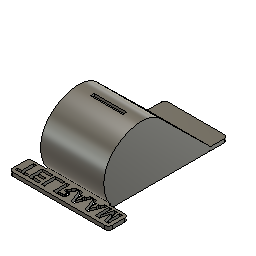
telraam_camera_holder_V1 (Autodesk Fusion 360 design; units mm, degrees)
Autodesk Fusion 360 part; units mm, degrees
note: some values were not read from the file. Chosen so that the rebuilt part matches the saved one: which bodies a step acts on; which face or edge a step refers to. Set by a fixed rule: which sketch regions a step uses.
sketch "Sketch1" plane through (0, 0, 0) normal (0, 1, 0) x (1, 0, 0)
  line L0 (0, 0) -> (30, 0)
  line L1 (30, 0) -> (30, 22)
  line L2 (30, 22) -> (0, 22)
  line L3 (0, 22) -> (0, 0)
  line L4 (0, 22) -> (2.25, 22) construction
  line L5 (2.25, 22) -> (2.25, 19.4) construction
  line L6 (2.25, 19.4) -> (0, 19.4) construction
  line L7 (0, 19.4) -> (0, 22) construction
  line L8 (2.25, 19.4) -> (27.75, 19.4)
  line L9 (27.75, 19.4) -> (27.75, -5)
  line L10 (27.75, -5) -> (2.25, -5)
  line L11 (2.25, -5) -> (2.25, 19.4)
  line L12 (15, -5) -> (15, 0) construction
  line L13 (15, 0) -> (22, 0) construction
  line L14 (22, 0) -> (8, 0)
  line L15 (8, 0) -> (8, 17.5)
  line L16 (8, 17.5) -> (22, 17.5)
  line L17 (22, 17.5) -> (22, 0)
  line L18 (30, 0) -> (0, 0)
  line L19 (0, 0) -> (0, -10)
  line L20 (0, -10) -> (30, -10)
  line L21 (30, -10) -> (30, 0)
  dimension "d1" = 30
  dimension "d2" = 22
  dimension "d3" = 2.25
  dimension "d4" = 2.6
  dimension "d5" = 25.5
  dimension "d6" = 24.4
  dimension "d7" = 5
  dimension "d8" = 7
  dimension "d9" = 14
  dimension "d10" = 17.5
  constraint horizontal L0
  constraint vertical L1
  constraint horizontal L2
  constraint vertical L3
  constraint coincident L0.start L3.end
  constraint horizontal L4
  constraint vertical L5
  constraint horizontal L6
  constraint vertical L7
  constraint horizontal L8
  constraint vertical L9
  constraint horizontal L10
  constraint vertical L11
  constraint midpoint L10 L12.start
  constraint perpendicular L10 L12
  constraint perpendicular L12 L13
  constraint horizontal L14
  constraint vertical L15
  constraint horizontal L16
  constraint vertical L17
  constraint horizontal L18
  constraint vertical L19
  constraint horizontal L20
  constraint vertical L21
  measures "d1" distance of L0.start L0.end
  measures "d2" distance of L0.start L2.end
  measures "d3" distance of L2.end L4.end
  measures "d4" distance of L2.end L6.end
  measures "d5" distance of L5.end L8.end
  measures "d6" distance of L5.end L10.end
  measures "d7" distance of L12.start L12.end
  measures "d8" distance of L12.end L13.end
  measures "d9" distance of L13.end L14.end
  measures "d10" distance of L13.end L16.end
extrude "Extrude1" add sketch "Sketch1" along normal blind 10 contours L0 L9 L10 L11 L18 L19 L20 L21 | L0 L1 L2 L3 L8 L9 L11 L18 makes body 1
extrude "Extrude2" add sketch "Sketch1" along normal blind 8 contours L0 L9 L10 L11 L14 L18 | L0 L8 L9 L11 L15 L16 L17 L18 bodies 1
sketch "Sketch2" plane through (0, 10, 0) normal (0, 1, 0) x (-1, 0, 0)
  line L0 (-27.75, 5) -> (-2.25, 5)
  line L1 (-2.25, 5) -> (-2.25, -19.4)
  line L2 (-2.25, -19.4) -> (-27.75, -19.4)
  line L3 (-27.75, -19.4) -> (-27.75, 5)
  line L4 (-30, 10) -> (-30, -22)
  line L5 (-30, -22) -> (0, -22)
  line L6 (0, -22) -> (0, 10)
  line L7 (0, 10) -> (-30, 10)
  line L8 (-15, 5) -> (-23.4414, 5) construction
  line L9 (-23.4414, 5) -> (-6.4414, 5)
  line L10 (-6.4414, 5) -> (-6.4414, 18)
  line L11 (-6.4414, 18) -> (-23.4414, 18)
  line L12 (-23.4414, 18) -> (-23.4414, 5)
  dimension "d15" = 17
  constraint midpoint L0 L8.start
  constraint coincident L0 L8.end
  constraint parallel L0 L8
  constraint horizontal L9
  constraint vertical L10
  constraint horizontal L11
  constraint vertical L12
  measures "d15" distance of L8.end L9.end
extrude "Extrude3" cut sketch "Sketch2" against normal blind 1 contours L0 L7 L9 L10 L12 bodies 1
sketch "Sketch5" plane through (0, 0, 0) normal (-1, 0, 0) x (0, 0, 1)
  line L0 (-22, 0) -> (10, 0)
  line L1 (10, 0) -> (10, 10)
  line L2 (10, 10) -> (-22, 10)
  line L3 (-22, 10) -> (-22, 0)
  line L4 (10, 10) -> (-22, 10)
  line L5 (10, 0) -> (10, 10)
  line L6 (-22, 0) -> (-22, 10)
  line L7 (10, 0) -> (-22, 0)
  line L8 (10, 5) -> (5, 5) construction
  circle A0 centre (5, 5) radius 5
  circle A1 centre (5, 5) radius 3
  dimension "d31" = 5
  dimension "d32" = 6
  constraint midpoint L1 L8.start
  constraint perpendicular L1 L8
  constraint coincident L8.end A0.centre
  constraint coincident L8.start A0
  constraint concentric A0 A1
  measures "d31" distance of L8.start L8.end
  measures "d32" diameter of A1
extrude "Extrude5" cut sketch "Sketch5" against normal blind 30 contours A1 bodies 1
extrude "Extrude6" cut sketch "Sketch5" against normal blind 30 contours L0 L1 L5 L7 A0 | L1 L2 L4 L5 A0 bodies 1
sketch "Sketch10" plane through (30, 0, 0) normal (1, 0, 0) x (0, 0, -1)
  arc A0 (-5, 10) -> (-5, 0) centre (-5, 5) ccw
  line L0 (-5, 0) -> (22, 0)
  line L1 (22, 0) -> (22, 10)
  line L2 (22, 10) -> (-5, 10)
  circle A1 centre (-5, 5) radius 3
  arc A2 (-5, 10) -> (-5, 0) centre (-5, 5) ccw
  circle A3 centre (-5, 5) radius 3
  line L3 (22, 10) -> (-5, 10)
  line L4 (22, 0) -> (22, 10)
  line L5 (22, 0) -> (-5, 0)
  circle A4 centre (-5, 5) radius 2.75
  circle A5 centre (-5, 5) radius 28 construction
  line L6 (-5, 5) -> (16.3152, 26.3152) construction
  line L7 (-5, 5) -> (25.7881, 5) construction
  line L8 (14.799, 24.799) -> (11.2635, 28.3345) construction
  line L9 (11.2635, 28.3345) -> (39.6303, -0.0323)
  line L10 (39.6303, -0.0323) -> (49.6303, -0.0323)
  spline S0 degree 5 poles (11.2635, 28.3345) (10.5414, 28.9553) (9.0442, 30.055) (6.6392, 31.2791) (3.1553, 32.0787) (-1.4187, 31.8066) (-5.8903, 30.427) (-9.919, 28.1364) (-13.2046, 25.151) (-15.548, 21.6967) (-16.9173, 18.001) (-17.397, 14.2819) (-17.1414, 10.738) (-16.3304, 7.5364) (-15.1311, 4.8024) (-13.6528, 2.6017) (-12.2918, 1.2849) (-11.1808, 0.5463) (-10.4002, 0.1638) (-10, 0) knots 0 0 0 0 0 0 0.066667 0.133333 0.2 0.266667 0.333333 0.4 0.466667 0.533333 0.6 0.666667 0.733333 0.8 0.866667 0.933333 1 1 1 1 1 1
  line L11 (15.5269, 24.669) -> (7, 32)
  spline S1 degree 5 poles (11.4377, 30.0185) (10.7333, 30.6009) (9.2645, 31.631) (6.8809, 32.7721) (3.3818, 33.5028) (-1.2891, 33.2032) (-5.9391, 31.8407) (-10.2242, 29.5954) (-13.8317, 26.6674) (-16.5299, 23.2679) (-18.243, 19.6138) (-19.051, 15.9194) (-19.1227, 12.3855) (-18.6719, 9.1891) (-17.9107, 6.4719) (-17.0026, 4.3263) (-16.2218, 3.0932) (-15.6179, 2.4413) (-15.2073, 2.127) (-15, 2) knots 0 0 0 0 0 0 0.066667 0.133333 0.2 0.266667 0.333333 0.4 0.466667 0.533333 0.6 0.666667 0.733333 0.8 0.866667 0.933333 1 1 1 1 1 1
  line L12 (15.4746, 26.6807) -> (7.4008, 33.3564)
  line L13 (-10, 0) -> (-25, 0)
  line L14 (-25, 0) -> (-25, 2)
  line L15 (-25, 2) -> (-15, 2)
  line L16 (49.6303, -0.0323) -> (49.6303, 1.9677)
  line L17 (49.6303, 1.9677) -> (40, 1.9677)
  line L18 (40, 1.9677) -> (11.4377, 30.0185)
  line L19 (-10, 0) -> (39.6303, -0.0323)
  point P0 (-13, 25)
  point P1 (-16, 7)
  point P2 (-15, 25)
  point P3 (-18, 7)
  dimension "d59" = 5.5
  dimension "d60" = 56
  dimension "d61" = 45
  dimension "d62" = 5
  dimension "d63" = 10
  dimension "d64" = 2
  constraint concentric A2 A4
  constraint concentric A4 A5
  constraint horizontal L7
  constraint coincident A0.centre A1.centre
  constraint coincident A5 L8.start
  constraint coincident L6 L8.start
  constraint perpendicular L6 L8
  constraint perpendicular L6 L9
  constraint horizontal L10
  constraint midpoint L8.end L11
  constraint midpoint S1.start L12
  constraint horizontal L13
  constraint perpendicular L13 L14
  constraint perpendicular L14 L15
  constraint perpendicular L10 L16
  constraint perpendicular L16 L17
  measures "d59" diameter of A4
  measures "d60" diameter of A5
  measures "d61" angle of L6 L7
  measures "d62" distance of L8.start L8.end
  measures "d63" distance of L9.end L10.end
  measures "d64" distance of L10.end L16.end
extrude "Extrude10" add sketch "Sketch10" along normal blind 2 from surface at 0.5 separate body contours A0 L0 L1 L2 A2 L3 L4 L5 | A1 A3 | A4 | L9 L10 S0 S1 L13 L14 L15 L16 L17 L18 | L9 S0 L19 makes body 2
extrude "Extrude11" add sketch "Sketch10" along normal blind -27 and the other way blind -1 contours A4 bodies 2
extrude "Extrude12" add sketch "Sketch10" along normal blind -30.5 and the other way blind -1 contours L9 L10 S0 S1 L13 L14 L15 L16 L17 L18 bodies 2
extrude "Extrude13" add sketch "Sketch10" against normal blind 2 from surface at -30.5 contours A0 L0 L1 L2 A2 L3 L4 L5 | A1 A3 | A4 | L9 L10 S0 S1 L13 L14 L15 L16 L17 L18 | L9 S0 L19 bodies 2
sketch "Sketch11" plane through (-2.5, 0, 0) normal (-1, 0, 0) x (0, 0, 1)
  line L0 (10, 0) -> (25, 0)
  line L1 (25, 0) -> (25, 2)
  line L2 (25, 2) -> (15, 2)
  spline S0 degree 5 poles (15, 2) (15.2073, 2.127) (15.6179, 2.4413) (16.2218, 3.0932) (17.0026, 4.3263) (17.9107, 6.4719) (18.6719, 9.1891) (19.1227, 12.3855) (19.051, 15.9194) (18.243, 19.6138) (16.5299, 23.2679) (13.8317, 26.6674) (10.2242, 29.5954) (5.9391, 31.8407) (1.2891, 33.2032) (-3.3818, 33.5028) (-6.8809, 32.7721) (-9.2645, 31.631) (-10.7333, 30.6009) (-11.4377, 30.0185) knots -1 -1 -1 -1 -1 -1 -0.933333 -0.866667 -0.8 -0.733333 -0.666667 -0.6 -0.533333 -0.466667 -0.4 -0.333333 -0.266667 -0.2 -0.133333 -0.066667 0 0 0 0 0 0
  line L3 (-11.4377, 30.0185) -> (-40, 1.9677)
  line L4 (-40, 1.9677) -> (-49.6303, 1.9677)
  line L5 (-49.6303, 1.9677) -> (-49.6303, -0.0323)
  line L6 (-49.6303, -0.0323) -> (-39.6303, -0.0323)
  line L7 (-39.6303, -0.0323) -> (10, 0)
  arc A0 (5, 0) -> (5, 10) centre (5, 5) ccw
  line L8 (5, 10) -> (-22, 10)
  circle A1 centre (5, 5) radius 3
  line L9 (-22, 0) -> (-22, 10)
  line L10 (5, 0) -> (-22, 0)
  circle A2 centre (5, 5) radius 5.5
  dimension "d79" = 11
  constraint concentric A0 A2
  measures "d79" diameter of A2
extrude "Extrude14" cut sketch "Sketch11" against normal blind 2 contours L7 L10 A2 | L7 A0 L8 A2 | L7 A0 L8 L10 A2 | A1 bodies 2
sketch "Sketch12" plane through (0, 0, 0) normal (-1, 0, 0) x (0, 0, 1)
  circle A0 centre (5, 5) radius 3
  arc A1 (5, 0) -> (5, 10) centre (5, 5) ccw
  line L0 (5, 10) -> (-22, 10)
  line L1 (-22, 10) -> (-22, 0)
  line L2 (-22, 0) -> (5, 0)
  circle A2 centre (5, 5) radius 5
  constraint concentric A0 A2
extrude "Extrude15" add sketch "Sketch12" along normal blind 3 contours A0 | A1 A2 bodies 1
sketch "Sketch13" plane through (-3, 0, 0) normal (-1, 0, 0) x (0, 0, 1)
  circle A0 centre (5, 5) radius 5
  line L0 (5, 0) -> (-22, 0)
  line L1 (-22, 0) -> (-22, 5)
  line L2 (-22, 5) -> (5, 5)
  line L3 (5, 5) -> (5, 0)
  constraint horizontal L0
  constraint vertical L1
  constraint horizontal L2
  constraint vertical L3
  constraint coincident A0 L0.start
extrude "Extrude16" add sketch "Sketch13" along normal blind 3 bodies 1
sketch "Sketch14" plane through (0, 0, 5) normal (0, 0, -1) x (-1, 0, 0)
  line L0 (-23.4414, 9) -> (-23.4414, 10)
  line L1 (-23.4414, 10) -> (-27.75, 10)
  line L2 (-27.75, 10) -> (-27.75, 8)
  line L3 (-27.75, 8) -> (-2.25, 8)
  line L4 (-2.25, 8) -> (-2.25, 10)
  line L5 (-2.25, 10) -> (-6.4414, 10)
  line L6 (-6.4414, 10) -> (-6.4414, 9)
  line L7 (-6.4414, 9) -> (-23.4414, 9)
  line L8 (-27.75, 10) -> (-26.8336, 10)
  line L9 (-26.8336, 10) -> (-26.8336, 9.2)
  line L10 (-26.8336, 9.2) -> (-27.75, 9.2)
  line L11 (-27.75, 9.2) -> (-27.75, 10)
  line L12 (-2.25, 10) -> (-3.1585, 10)
  line L13 (-3.1585, 10) -> (-3.1585, 9.2)
  line L14 (-3.1585, 9.2) -> (-2.25, 9.2)
  line L15 (-2.25, 9.2) -> (-2.25, 10)
  dimension "d88" = 0.8
  dimension "d89" = 0.8
  constraint horizontal L8
  constraint vertical L9
  constraint horizontal L10
  constraint vertical L11
  constraint coincident L1.end L2.start
  constraint horizontal L12
  constraint vertical L13
  constraint horizontal L14
  constraint vertical L15
  constraint coincident L4.end L5.start
  measures "d88" distance of L1.end L10.end
  measures "d89" distance of L4.end L14.end
extrude "Extrude17" add sketch "Sketch14" along normal blind 2 contours L1 L2 L8 L9 L10 L11 | L4 L5 L12 L13 L14 L15 bodies 1
fillet "Fillet5" radius 0.5 4 edges at (3.1585, 9.2, 4) (2.7043, 9.2, 3) (26.8336, 9.2, 4) (27.2918, 9.2, 3) on bodies 1
sketch "Sketch15" plane through (0, 0, -19.4) normal (0, 0, 1) x (1, 0, 0)
  line L0 (2.25, 8) -> (27.75, 8)
  line L1 (27.75, 8) -> (27.75, 10)
  line L2 (27.75, 10) -> (2.25, 10)
  line L3 (2.25, 10) -> (2.25, 8)
  line L4 (9.9542, 10) -> (20.0929, 10)
  line L5 (20.0929, 10) -> (20.0929, 9.2)
  line L6 (20.0929, 9.2) -> (9.9542, 9.2)
  line L7 (9.9542, 9.2) -> (9.9542, 10)
  dimension "d94" = 0.8
  constraint horizontal L4
  constraint vertical L5
  constraint horizontal L6
  constraint vertical L7
  constraint coincident L2 L4.start
  measures "d94" distance of L4.start L6.end
extrude "Extrude18" add sketch "Sketch15" along normal blind 0.4 contours L2 L4 L5 L6 L7 bodies 1
fillet "Fillet6" radius 0.4 2 edges at (15.0235, 10, -19) (15.0235, 9.2, -19) on bodies 1
fillet "Fillet7" radius 4 2 edges at (30, 5, -22) (0, 5, -22) on bodies 1
sketch "Sketch17" plane through (0, 0, 0) normal (0, 1, 0) x (1, 0, 0)
  arc A0 (4, 22) -> (0, 18) centre (4, 18) ccw
  line L0 (26, 22) -> (4, 22)
  arc A1 (30, 18) -> (26, 22) centre (26, 18) ccw
  line L1 (30, -10) -> (30, -5)
  line L2 (30, -5) -> (30, 18)
  line L3 (-3, 0) -> (-3, 22)
  line L4 (-6, 22) -> (-6, -5)
  line L5 (-3, 22) -> (-6, 22)
  line L6 (-6, -5) -> (-6, -10)
  line L7 (0, 18) -> (0, 0)
  line L8 (8, 0) -> (8, 17.5)
  line L9 (22, 0) -> (8, 0)
  line L10 (22, 17.5) -> (22, 0)
  line L11 (8, 17.5) -> (22, 17.5)
  line L12 (-6, -10) -> (30, -10)
  line L13 (-3, 0) -> (0, 0)
  line L14 (6, 0) -> (24, 0)
  line L15 (24, 0) -> (24, 2)
  line L16 (24, 2) -> (6, 2)
  line L17 (6, 2) -> (6, 0)
  constraint horizontal L14
  constraint vertical L15
  constraint horizontal L16
  constraint vertical L17
extrude "Extrude19" cut sketch "Sketch17" along normal blind 37 from surface at 20 contours L8 L14 L16 L17 | L8 L9 L10 L14 L16 | L10 L14 L15 L16 bodies 2
sketch "Sketch18" plane through (0, 0, 0) normal (0, -1, 0) x (1, 0, 0)
  line L0 (-2.5, 25) -> (-2.5, 10)
  line L1 (-2.5, 10) -> (-0.5, 10)
  line L2 (-0.5, 10) -> (30.5, 10)
  line L3 (30.5, 10) -> (32.5, 10)
  line L4 (32.5, 10) -> (32.5, 25)
  line L5 (32.5, 25) -> (-2.5, 25)
  line L6 (-10.5777, 8.9762) -> (41.4223, 8.9762) construction
  line L7 (41.4223, 8.9762) -> (41.4223, 24.9762) construction
  line L8 (41.4223, 24.9762) -> (-10.5777, 24.9762) construction
  line L9 (-10.5777, 24.9762) -> (-10.5777, 8.9762) construction
  line L10 (-12, 16) -> (43, 16)
  line L11 (43, 16) -> (43, 27)
  line L12 (43, 27) -> (-12, 27)
  line L13 (-12, 27) -> (-12, 16)
  line L14 (12.2105, 23.7055) -> (9.3109, 23.7055)
  line L15 (9.3109, 23.7055) -> (9.3109, 21.8124)
  line L16 (9.3109, 21.8124) -> (12.2105, 21.8124)
  line L17 (12.2105, 21.8124) -> (12.2105, 23.7055)
  line L18 (20.5, 20.5) -> (21.6042, 20.5)
  line L19 (21.6042, 20.5) -> (21.6042, 18.745)
  line L20 (21.6042, 18.745) -> (20.5, 18.745)
  line L21 (20.5, 18.745) -> (20.5, 20.5)
  line L22 (28.2661, 20.5) -> (29.3444, 20.5)
  line L23 (29.3444, 20.5) -> (29.3444, 18.745)
  line L24 (29.3444, 18.745) -> (28.2661, 18.745)
  line L25 (28.2661, 18.745) -> (28.2661, 20.5)
  point P0 (15, 25)
  text T0 "TELRAAM" font "Arial" height 7.7 bold align left top in box 52 x 16 at (-10.5777, 8.9762) x (1, 0) y (0, 1) spacing 1
  constraint midpoint L5 P0
  constraint horizontal L10
  constraint vertical L11
  constraint horizontal L12
  constraint vertical L13
  constraint horizontal L14
  constraint vertical L15
  constraint horizontal L16
  constraint vertical L17
  constraint horizontal L18
  constraint vertical L19
  constraint horizontal L20
  constraint vertical L21
  constraint horizontal L22
  constraint vertical L23
  constraint horizontal L24
  constraint vertical L25
extrude "Extrude20" add sketch "Sketch18" against normal blind 2 contours L0 L4 L5 L10 L11 L12 L13 bodies 2
extrude "Extrude22" cut sketch "Sketch18" against normal blind 2 text T0 bodies 2 makes body 3 at (12.6379, 2, 23.0223) makes body 4 at (29.554, 0.6667, 21.275) makes body 5 at (21.7858, 0.6667, 21.275)
sketch "Sketch19" plane through (0, 2, 0) normal (0, 1, 0) x (-1, 0, 0)
  line L0 (-32.5, 16) -> (-32.5, 15)
  line L1 (-32.5, 15) -> (2.5, 15)
  line L2 (2.5, 15) -> (2.5, 16)
  line L3 (2.5, 16) -> (12, 16)
  line L4 (12, 16) -> (12, 27)
  line L5 (12, 27) -> (-43, 27)
  line L6 (-43, 27) -> (-43, 16)
  line L7 (-43, 16) -> (-32.5, 16)
  line L8 (6.7382, 17.2762) -> (6.7382, 23.6736)
  line L9 (6.7382, 23.6736) -> (4.4587, 23.6736)
  line L10 (4.4587, 23.6736) -> (4.4587, 24.9762)
  line L11 (4.4587, 24.9762) -> (10.5777, 24.9762)
  line L12 (10.5777, 24.9762) -> (10.5777, 23.6736)
  line L13 (10.5777, 23.6736) -> (8.2929, 23.6736)
  line L14 (8.2929, 23.6736) -> (8.2929, 17.2762)
  line L15 (8.2929, 17.2762) -> (6.7382, 17.2762)
  line L16 (-9.1818, 17.2762) -> (-9.1818, 18.5735)
  line L17 (-9.1818, 18.5735) -> (-5.316, 18.5735)
  line L18 (-5.316, 18.5735) -> (-5.316, 24.9132)
  line L19 (-5.316, 24.9132) -> (-3.7613, 24.9132)
  line L20 (-3.7613, 24.9132) -> (-3.7613, 17.2762)
  line L21 (-3.7613, 17.2762) -> (-9.1818, 17.2762)
  line L22 (-11.85, 17.2762) -> (-11.85, 20.4906)
  line L23 (-11.85, 20.4906) -> (-12.1651, 20.4906)
  spline S0 degree 3 poles (-12.1651, 20.4906) (-12.3206, 20.4903) (-12.5852, 20.4898) (-12.8418, 20.4272) (-12.9477, 20.4014) knots -0.07901 -0.07901 -0.07901 -0.07901 -0.032603 0 0 0 0
  spline S1 degree 3 poles (-12.9477, 20.4014) (-13.0308, 20.365) (-13.2067, 20.2879) (-13.3432, 20.1525) (-13.4152, 20.081) knots -0.057107 -0.057107 -0.057107 -0.057107 -0.030153 0 0 0 0
  spline S2 degree 3 poles (-13.4152, 20.081) (-13.5219, 19.9495) (-13.8153, 19.5881) (-14.0715, 19.1992) (-14.2346, 18.9517) knots -0.139592 -0.139592 -0.139592 -0.139592 -0.088836 0 0 0 0
  line L24 (-14.2346, 18.9517) -> (-15.3586, 17.2762)
  line L25 (-15.3586, 17.2762) -> (-17.2179, 17.2762)
  line L26 (-17.2179, 17.2762) -> (-16.2778, 18.7784)
  spline S3 degree 3 poles (-16.2778, 18.7784) (-16.1175, 19.0369) (-15.8476, 19.4724) (-15.5223, 19.8678) (-15.3901, 20.0284) knots -0.153464 -0.153464 -0.153464 -0.153464 -0.062342 0 0 0 0
  spline S4 degree 3 poles (-15.3901, 20.0284) (-15.2703, 20.1455) (-15.0181, 20.392) (-14.7178, 20.5772) (-14.5602, 20.6745) knots -0.105457 -0.105457 -0.105457 -0.105457 -0.055357 0 0 0 0
  spline S5 degree 3 poles (-14.5602, 20.6745) (-14.8687, 20.7321) (-15.4392, 20.8386) (-15.8806, 21.212) (-16.0834, 21.3836) knots -0.170594 -0.170594 -0.170594 -0.170594 -0.078353 0 0 0 0
  spline S6 degree 3 poles (-16.0834, 21.3836) (-16.232, 21.5899) (-16.54, 22.0177) (-16.5748, 22.5447) (-16.5929, 22.8175) knots -0.154918 -0.154918 -0.154918 -0.154918 -0.080198 0 0 0 0
  spline S7 degree 3 poles (-16.5929, 22.8175) (-16.5802, 23.0367) (-16.5553, 23.4655) (-16.3548, 23.8452) (-16.2568, 24.0308) knots -0.127215 -0.127215 -0.127215 -0.127215 -0.062196 0 0 0 0
  spline S8 degree 3 poles (-16.2568, 24.0308) (-16.1366, 24.1935) (-15.8993, 24.5149) (-15.5372, 24.6831) (-15.3586, 24.7661) knots -0.117747 -0.117747 -0.117747 -0.117747 -0.058096 0 0 0 0
  spline S9 degree 3 poles (-15.3586, 24.7661) (-15.1176, 24.8269) (-14.5309, 24.9749) (-13.9248, 24.9757) (-13.5675, 24.9762) knots -0.180926 -0.180926 -0.180926 -0.180926 -0.106622 0 0 0 0
  line L27 (-13.5675, 24.9762) -> (-10.2953, 24.9762)
  line L28 (-10.2953, 24.9762) -> (-10.2953, 17.2762)
  line L29 (-10.2953, 17.2762) -> (-11.85, 17.2762)
  line L30 (-29.6871, 24.9762) -> (-28.0431, 24.9762)
  line L31 (-28.0431, 24.9762) -> (-25.044, 17.2762)
  line L32 (-25.044, 17.2762) -> (-26.6932, 17.2762)
  line L33 (-26.6932, 17.2762) -> (-27.3288, 19.0252)
  line L34 (-27.3288, 19.0252) -> (-30.4067, 19.0252)
  line L35 (-30.4067, 19.0252) -> (-31.079, 17.2762)
  line L36 (-31.079, 17.2762) -> (-32.7703, 17.2762)
  line L37 (-32.7703, 17.2762) -> (-29.6871, 24.9762)
  line L38 (-21.9188, 24.9762) -> (-20.2748, 24.9762)
  line L39 (-20.2748, 24.9762) -> (-17.2757, 17.2762)
  line L40 (-17.2757, 17.2762) -> (-18.925, 17.2762)
  line L41 (-18.925, 17.2762) -> (-19.5605, 19.0252)
  line L42 (-19.5605, 19.0252) -> (-22.6384, 19.0252)
  line L43 (-22.6384, 19.0252) -> (-23.3107, 17.2762)
  line L44 (-23.3107, 17.2762) -> (-25.002, 17.2762)
  line L45 (-25.002, 17.2762) -> (-21.9188, 24.9762)
  line L46 (-35.0183, 17.2762) -> (-35.0183, 23.3374)
  line L47 (-35.0183, 23.3374) -> (-36.5415, 17.2762)
  line L48 (-36.5415, 17.2762) -> (-38.0384, 17.2762)
  line L49 (-38.0384, 17.2762) -> (-39.5669, 23.3374)
  line L50 (-39.5669, 23.3374) -> (-39.5669, 17.2762)
  line L51 (-39.5669, 17.2762) -> (-41.0113, 17.2762)
  line L52 (-41.0113, 17.2762) -> (-41.0113, 24.9762)
  line L53 (-41.0113, 24.9762) -> (-38.6792, 24.9762)
  line L54 (-38.6792, 24.9762) -> (-37.2978, 19.7238)
  line L55 (-37.2978, 19.7238) -> (-35.9007, 24.9762)
  line L56 (-35.9007, 24.9762) -> (-33.5739, 24.9762)
  line L57 (-33.5739, 24.9762) -> (-33.5739, 17.2762)
  line L58 (-33.5739, 17.2762) -> (-35.0183, 17.2762)
  line L59 (-2.401, 17.2762) -> (-2.401, 18.5735)
  line L60 (-2.401, 18.5735) -> (1.9007, 18.5735)
  line L61 (1.9007, 18.5735) -> (1.9007, 20.6692)
  line L62 (1.9007, 20.6692) -> (-1.965, 20.6692)
  line L63 (-1.965, 20.6692) -> (-1.965, 21.9666)
  line L64 (-1.965, 21.9666) -> (1.9007, 21.9666)
  line L65 (1.9007, 21.9666) -> (1.9007, 23.6736)
  line L66 (1.9007, 23.6736) -> (-2.2539, 23.6736)
  line L67 (-2.2539, 23.6736) -> (-2.2539, 24.9762)
  line L68 (-2.2539, 24.9762) -> (3.4555, 24.9762)
  line L69 (3.4555, 24.9762) -> (3.4555, 17.2762)
  line L70 (3.4555, 17.2762) -> (-2.401, 17.2762)
  line L71 (-11.85, 21.8295) -> (-13.1477, 21.8295)
  line L72 (-13.1477, 21.8295) -> (-13.1477, 20.3044)
  line L73 (-13.1477, 20.3044) -> (-11.85, 20.3044)
  line L74 (-11.85, 20.3044) -> (-11.85, 21.8295)
  line L75 (-21.6279, 20.4295) -> (-20.5016, 20.4295)
  line L76 (-20.5016, 20.4295) -> (-20.5016, 18.5544)
  line L77 (-20.5016, 18.5544) -> (-21.6279, 18.5544)
  line L78 (-21.6279, 18.5544) -> (-21.6279, 20.4295)
  line L79 (-29.4763, 20.429) -> (-28.3136, 20.429)
  line L80 (-28.3136, 20.429) -> (-28.3136, 19.0252)
  line L81 (-28.3136, 19.0252) -> (-29.4763, 19.0252)
  line L82 (-29.4763, 19.0252) -> (-29.4763, 20.429)
  constraint horizontal L71
  constraint vertical L72
  constraint horizontal L73
  constraint vertical L74
  constraint coincident S1 L72.end
  constraint horizontal L75
  constraint vertical L76
  constraint horizontal L77
  constraint vertical L78
  constraint horizontal L79
  constraint vertical L80
  constraint horizontal L81
  constraint vertical L82
  constraint coincident L34 L80.end
extrude "Extrude23" add sketch "Sketch19" against normal blind 2 contours L23 S0 S1 L71 L72 L74 | L34 L79 L80 L81 L82 | L42 L75 L76 L78 bodies 2
combine "Combine2" operation add target body 2 tool bodies 3 4 5
fillet "Fillet8" radius 2 6 edges at (-2.5, 0.9677, -49.6303) (43, 1, 16) (43, 1, 27) (-12, 1, 27) (-12, 1, 16) (32.5, 0.9677, -49.6303) on bodies 2
